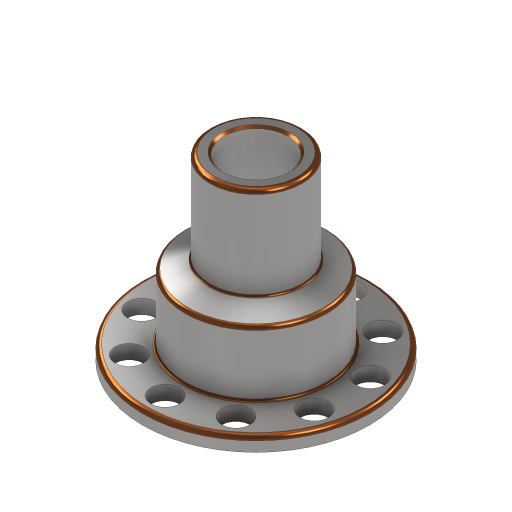
# Autodesk Inventor part: Brida
Saved by Autodesk Inventor 2023 (Build 270158000, 158)
## iProperties
Created: 2023-04-12
Part Number: Brida
Material: Acero, fundido
Document SubType Name: Modeling
Designer: JUAN
Density: 7.85 g/cm^3
Appearance: Semipulido
Mass: 24871.6 g
Surface Area: 3616.17 cm^2
Volume: 3168.36 cm^3
Author: JUAN
Autodesk Inventor part; units mm, degrees
ref_plane "YZ Plane" through (0, 0, 0) normal (1, 0, 0) x (0, 1, 0)
ref_plane "XZ Plane" through (0, 0, 0) normal (0, 1, 0) x (-1, 0, 0)
ref_plane "XY Plane" through (0, 0, 0) normal (0, 0, 1) x (1, 0, 0)
sketch "Boceto1" plane through (0, 0, 0) normal (1, 0, 0) x (0, 1, 0)
  line L0 (0, 0) -> (253.6364, 0) construction
  line L1 (253.6364, 45) -> (109.2844, 45)
  line L2 (109.2844, 45) -> (96.5455, 80)
  line L3 (96.5455, 80) -> (0, 80)
  line L4 (0, 80) -> (0, 160)
  line L5 (0, 160) -> (20, 160)
  line L6 (20, 160) -> (20, 100)
  line L7 (20, 100) -> (110.5496, 100)
  line L8 (110.5496, 100) -> (123.2886, 65)
  line L9 (253.6364, 45) -> (253.6364, 65)
  line L10 (253.6364, 65) -> (122.5163, 65)
  dimension "d0" = 45
  dimension "d1" = 160
  dimension "d2" = 80
  dimension "d3" = 20
  dimension "d4" = 20
  dimension "d7" = 20
  dimension "d8" = 20
  dimension "d9" = 110
  constraints: 22 end point, 5 perpendicular, 2 horizontal, 2 parallel, 1 point on line, 1 vertical
  measures "d0" distance between parallel lines of L0 L1
  measures "d1" distance between parallel lines of L0 L5
  measures "d2" distance between parallel lines of L0 L3
  measures "d3" distance between parallel lines of L2 L8
  measures "d4" distance between parallel lines of L4 L6
  measures "d7" distance between parallel lines of L3 L7
  measures "d8" distance between parallel lines of L1 L10
  measures "d9" angle of L8 L10
revolve "Revolución1" add sketch "Boceto1" angle 360 mid plane about axis through (0, 0, 0) along (0, 1, 0)
sketch "Boceto2" plane through (0, 20, 0) normal (0, 1, 0) x (1, 0, 0)
  circle A0 centre (0, 128) radius 20
  circle A1 centre (0, 0) radius 128 construction
  dimension "d12" = 256
  dimension "d11" = 40
  constraints: 1 centre point, 1 coincident, 1 vertical alignment, 2 other
  measures "d11" diameter of A0
extrude "Extrusión1" cut sketch "Boceto2" against normal through all
pattern_circular "Patrón circular1" count 10 over 360 about axis through (0, 181.4604, 0) along (0, 1, 0) of "Extrusión1"
fillet "Empalme1" radius 3 2 edges at (0, 20, 100) (0, 123.2886, 65)
fillet "Empalme2" radius 6 3 edges at (0, 110.5496, 100) (0, 253.6364, 65) (0, 20, 160)
fillet "Empalme3" radius 6 1 edges at (0, 96.5455, 80)
chamfer "Chaflán1" distance 6 angle 45 1 edges at (0, 0, 80)
chamfer "Chaflán2" distance 3 angle 45 1 edges at (0, 253.6364, 45)
